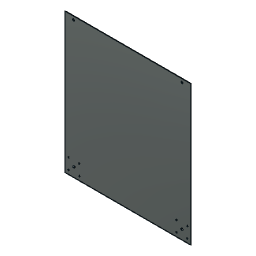
h_bot_Dec26 v12 (Autodesk Fusion 360 design; units mm, degrees)
Autodesk Fusion 360 part; units mm, degrees
sketch "Sketch2" plane through (0, 0, 0) normal (0, 0, 1) x (1, 0, 0)
  line L0 (0, 0) -> (553.4775, 0) construction
  line L1 (0, 0) -> (-537.9839, 0) construction
  line L2 (0, 0) -> (0, 375) construction
  line L3 (0, 0) -> (0, -800) construction
  line L4 (-180, 200) -> (180, 200)
  line L5 (180, 200) -> (180, -200)
  line L6 (180, -200) -> (-180, -200)
  line L7 (-180, -200) -> (-180, 200)
  line L8 (-170, -157.8089) -> (-139, -188.8089) construction
  line L9 (-139, -157.8089) -> (-170, -188.8089) construction
  line L10 (139, -158.0835) -> (170, -189.0835) construction
  line L11 (170, -158.0835) -> (139, -189.0835) construction
  circle A0 centre (-154.5, -173.3089) radius 8
  circle A1 centre (154.5, -173.5835) radius 8
  circle A2 centre (139, -158.0835) radius 1.75
  circle A3 centre (139, -189.0835) radius 1.75
  circle A4 centre (170, -189.0835) radius 1.75
  circle A5 centre (170, -158.0835) radius 1.75
  line L12 (-108, 159) -> (108, 159)
  line L13 (108, 159) -> (108, -120)
  line L14 (108, -120) -> (-108, -120)
  line L15 (-108, -120) -> (-108, 159)
  line L16 (154.5, -173.5835) -> (154.5, 269.9863) construction
  line L17 (-155.5, -173.9681) -> (-155.5, 269.9863) construction
  line L18 (-319.8669, 190) -> (350, 190) construction
  circle A6 centre (-155.5, 190) radius 11.5
  circle A7 centre (154.5, 190) radius 11.5
  circle A8 centre (-155.5, 190) radius 2.5
  circle A9 centre (154.5, 190) radius 2.5
  line L19 (-144, 190) -> (-144, -80) construction
  line L20 (143, 190) -> (143, -60) construction
  circle A10 centre (-170, -157.8089) radius 1.75
  circle A11 centre (-139, -157.8089) radius 1.75
  circle A12 centre (-170, -188.8089) radius 1.75
  circle A13 centre (-139, -188.8089) radius 1.75
  circle A14 centre (-154.5, -173.3089) radius 2.75
  circle A15 centre (154.5, -173.5835) radius 2.75
  point P0 (-170, -188.8089)
  point P1 (-139, -188.8089)
  point P2 (-139, -157.8089)
  point P3 (-170, -157.8089)
  point P4 (125, -200)
  point P5 (170, -158.0835)
  point P6 (139, -189.0835)
  point P7 (139, -158.0835)
  point P8 (170, -189.0835)
  dimension "d11" = 360
  dimension "d12" = 400
  dimension "d36" = 31
  dimension "d37" = 31
  dimension "d38" = 10
  dimension "d39" = 31
  dimension "d40" = 31
  dimension "d41" = 10
  dimension "d42" = 16
  dimension "d43" = 16
  dimension "d44" = 3.5
  dimension "d46" = 3.5
  dimension "d47" = 3.5
  dimension "d48" = 3.5
  dimension "d49" = 279
  dimension "d50" = 216
  dimension "d51" = 80
  dimension "d52" = 10
  dimension "d53" = 23
  dimension "d54" = 23
  dimension "d55" = 5
  dimension "d56" = 5
  dimension "d57" = 24.5
  dimension "d68" = 3.5
  dimension "d69" = 3.5
  dimension "d70" = 3.5
  dimension "d71" = 3.5
  dimension "d72" = 5.5
  dimension "d73" = 5.5
  constraint coincident L0.start L1.start
  constraint horizontal L0
  constraint parallel L0 L1
  constraint perpendicular L0 L2
  constraint perpendicular L0 L3
  constraint horizontal L4
  constraint vertical L5
  constraint horizontal L6
  constraint vertical L7
  constraint symmetric L1 L4 L6
  constraint symmetric L2 L5 L7
  constraint vertical P1 P2
  constraint vertical P0 P3
  constraint horizontal P2 P3
  constraint horizontal P0 P1
  constraint coincident P3 L8.start
  constraint coincident P1 L8.end
  constraint coincident P2 L9.start
  constraint coincident P0 L9.end
  constraint vertical P5 P8
  constraint vertical P6 P7
  constraint horizontal P5 P7
  constraint horizontal P6 P8
  constraint coincident P7 L10.start
  constraint coincident P8 L10.end
  constraint coincident P5 L11.start
  constraint coincident P6 L11.end
  constraint midpoint L9 A0.centre
  constraint midpoint L10 A1.centre
  constraint horizontal L12
  constraint vertical L13
  constraint horizontal L14
  constraint vertical L15
  constraint symmetric L2 L13 L15
  constraint coincident A1.centre L16.start
  constraint perpendicular L4 L16
  constraint perpendicular L5 L18
  constraint coincident L18 A6.centre
  constraint coincident L17 A6.centre
  constraint coincident L18 A7.centre
  constraint coincident L16 A7.centre
  constraint concentric A6 A8
  constraint concentric A7 A9
  constraint coincident L18 L19.start
  constraint coincident A6 L19.start
  constraint tangent A6 L19
  constraint coincident L18 L20.start
  constraint coincident A7 L20.start
  constraint tangent A7 L20
  constraint concentric A0 A14
  constraint concentric A1 A15
  measures "d11" distance of L4.start L4.end
  measures "d12" distance of L4.end L5.end
  measures "d36" distance of P0 P1
  measures "d37" distance of P0 P3
  measures "d38" distance of L7 P0
  measures "d39" distance of P6 P8
  measures "d40" distance of P6 P7
  measures "d41" distance of L5 P8
  measures "d42" diameter of A0
  measures "d43" diameter of A1
  measures "d44" diameter of A2
  measures "d46" diameter of A3
  measures "d47" diameter of A4
  measures "d48" diameter of A5
  measures "d49" distance of L12.end L13.end
  measures "d50" distance of L12.start L12.end
  measures "d51" distance of L6 L14
  measures "d52" distance of L4 L18
  measures "d53" diameter of A6
  measures "d54" diameter of A7
  measures "d55" diameter of A8
  measures "d56" diameter of A9
  measures "d57" distance of L7 A6.centre
  measures "d68" diameter of A10
  measures "d69" diameter of A11
  measures "d70" diameter of A12
  measures "d71" diameter of A13
  measures "d72" diameter of A14
  measures "d73" diameter of A15
extrude "Extrude2" add sketch "Sketch2" along normal blind 6 contours L4 L5 L6 L7 A6 A7 | L4 A6 | L4 A7 | A0 | A1 | A2 | A3 | A4 | A5 | L12 L13 L14 L15 | A8 | A9 | A10 | A11 | A12 | A13 | A14 | A15 picked at (-155.5623, 197.4977) picked at (154.4377, 197.4977) makes body 1
sketch "Sketch3" plane through (0, 0, 6) normal (0, 0, 1) x (1, 0, 0)
  line L0 (-180, -200) -> (180, -200)
  line L1 (180, -200) -> (180, 200)
  line L2 (180, 200) -> (-180, 200)
  line L3 (-180, 200) -> (-180, -200)
  line L4 (-150, 37.5) -> (150, 37.5)
  line L5 (150, 37.5) -> (150, -37.5)
  line L6 (150, -37.5) -> (-150, -37.5)
  line L7 (-150, -37.5) -> (-150, 37.5)
  line L8 (0, 0) -> (553.4775, 0)
  line L9 (0, 0) -> (0, 375)
  line L10 (0, 0) -> (-537.9839, 0)
  line L11 (-125, 7.5) -> (125, 7.5)
  line L12 (125, 7.5) -> (125, -7.5)
  line L13 (125, -7.5) -> (-125, -7.5)
  line L14 (-125, -7.5) -> (-125, 7.5)
  circle A0 centre (-132.4183, 22.14) radius 11.5
  circle A1 centre (-132.4183, -22.14) radius 11.5
  circle A2 centre (132.4183, 22.14) radius 11.5
  circle A3 centre (132.4183, -22.14) radius 11.5
  line L15 (0, 0) -> (0, -800)
  circle A4 centre (-132.4183, 22.14) radius 2.5
  circle A5 centre (-132.4183, -22.14) radius 2.5
  circle A6 centre (132.4183, 22.14) radius 2.5
  circle A7 centre (132.4183, -22.14) radius 2.5
  dimension "d19" = 300
  dimension "d20" = 75
  dimension "d24" = 30
  dimension "d26" = 250
  dimension "d58" = 23
  dimension "d59" = 23
  dimension "d60" = 23
  dimension "d61" = 23
  dimension "d62" = 5
  dimension "d63" = 5
  dimension "d64" = 5
  dimension "d65" = 5
  constraint horizontal L4
  constraint vertical L5
  constraint horizontal L6
  constraint vertical L7
  constraint symmetric L4 L6 L8
  constraint symmetric L5 L7 L9
  constraint horizontal L11
  constraint vertical L12
  constraint horizontal L13
  constraint vertical L14
  constraint symmetric L8 L11 L13
  constraint symmetric L9 L12 L14
  constraint symmetric L10 A0 A1
  constraint symmetric L9 A0 A2
  constraint symmetric A1 A3 L15
  constraint concentric A0 A4
  constraint concentric A1 A5
  constraint concentric A2 A6
  constraint concentric A3 A7
  measures "d19" distance of L4.start L4.end
  measures "d20" distance of L4.end L5.end
  measures "d24" distance of L4 L11.start
  measures "d26" distance of L12 L14
  measures "d58" diameter of A0
  measures "d59" diameter of A1
  measures "d60" diameter of A2
  measures "d61" diameter of A3
  measures "d62" diameter of A4
  measures "d63" diameter of A5
  measures "d64" diameter of A6
  measures "d65" diameter of A7
extrude "Extrude3" add sketch "Sketch3" along normal blind 6 separate body contours L5 L6 L8 L12 L13 L15 | L6 L7 L10 L13 L14 L15 | L4 L7 L9 L10 L11 L14 | L4 L5 L8 L9 L11 L12 | A0 | A1 | A2 | A3 | A4 | A5 | A6 | A7 makes body 2
sketch "Sketch4" plane through (0, 0, 12) normal (0, 0, 1) x (1, 0, 0)
  line L0 (-125, -7.5) -> (-125, 7.5)
  line L1 (-125, 7.5) -> (125, 7.5)
  line L2 (125, 7.5) -> (125, -7.5)
  line L3 (-150, -37.5) -> (150, -37.5)
  line L4 (150, -37.5) -> (150, 37.5)
  line L5 (150, 37.5) -> (-150, 37.5)
  line L6 (-150, 37.5) -> (-150, -37.5)
  line L7 (9.5492, 18.75) -> (34.5492, 18.75)
  line L8 (34.5492, 18.75) -> (34.5492, -18.75)
  line L9 (34.5492, -18.75) -> (9.5492, -18.75)
  line L10 (9.5492, -18.75) -> (9.5492, 18.75)
  line L11 (0, 0) -> (-537.9839, 0)
  line L12 (125, -7.5) -> (-125, -7.5)
  dimension "d31" = 37.5
  dimension "d32" = 25
  constraint horizontal L7
  constraint vertical L8
  constraint horizontal L9
  constraint vertical L10
  constraint symmetric L7 L9 L11
  measures "d31" distance of L7.start L9.end
  measures "d32" distance of L8.end L9.end
extrude "Extrude5" add sketch "Sketch3" along normal blind 5 separate body contours L5 L6 L8 L12 L13 L15 | L6 L7 L10 L13 L14 L15 | L4 L7 L9 L10 L11 L14 | L4 L5 L8 L9 L11 L12 | A0 | A1 | A2 | A3 makes body 3
sketch "Sketch5" plane through (0, 0, 11) normal (0, 0, 1) x (1, 0, 0)
  circle A0 centre (-132.4183, 22.14) radius 2.5
  line L0 (125, -7.5) -> (-125, -7.5)
  line L1 (-125, -7.5) -> (-125, 7.5)
  line L2 (-125, 7.5) -> (125, 7.5)
  line L3 (125, 7.5) -> (125, -7.5)
  circle A1 centre (132.4183, 22.14) radius 2.5
  circle A2 centre (-132.4183, -22.14) radius 2.5
  circle A3 centre (132.4183, -22.14) radius 2.5
  line L4 (-150, -37.5) -> (150, -37.5)
  line L5 (150, -37.5) -> (150, 37.5)
  line L6 (150, 37.5) -> (-150, 37.5)
  line L7 (-150, 37.5) -> (-150, -37.5)
extrude "Extrude6" add sketch "Sketch2" along normal blind 1 separate body contours L4 L5 L6 L7 A6 A7 | L4 A6 | L4 A7 | A0 | A1 | L12 L13 L14 L15 picked at (-155.5623, 197.4977) picked at (154.4377, 197.4977) makes body 4
sketch "Sketch7" plane through (0, 0, 1) normal (0, 0, 1) x (1, 0, 0)
  circle A0 centre (-170, -157.8089) radius 1.75
  circle A1 centre (154.5, 190) radius 2.5
  circle A2 centre (154.5, -173.5835) radius 2.75
  circle A3 centre (-154.5, -173.3089) radius 2.75
  circle A4 centre (170, -189.0835) radius 1.75
  circle A5 centre (-155.5, 190) radius 2.5
  circle A6 centre (139, -189.0835) radius 1.75
  circle A7 centre (-170, -188.8089) radius 1.75
  circle A8 centre (-139, -157.8089) radius 1.75
  circle A9 centre (170, -158.0835) radius 1.75
  circle A10 centre (-139, -188.8089) radius 1.75
  circle A11 centre (139, -158.0835) radius 1.75
  line L0 (-180, -200) -> (180, -200)
  line L1 (180, -200) -> (180, 200)
  line L2 (180, 200) -> (-180, 200)
  line L3 (-180, 200) -> (-180, -200)
extrude "Extrude4" [rolled back] along distance 6 taper angle 0
hidden bodies 1 2 3
equation "frame_height = 400 mm"
equation "frame_width = 360 mm"
equation "frame_thickness = 40 mm"
equation "d11 = frame_width"
equation "d12 = frame_height"
equation "y_carriage_height = 75 mm"
equation "y_carriage_width = 300 mm"
equation "d19 = y_carriage_width"
equation "d20 = y_carriage_height"
equation "y_carriage_thickness = 30 mm"
equation "d24 = y_carriage_thickness"
equation "y_carriage_inner_width = 250 mm"
equation "d26 = y_carriage_inner_width"
equation "x_carriage_width = 25 mm"
equation "x_carriage_height = 25 mm"
equation "d31 = x_carriage_height * 1.5"
equation "d32 = x_carriage_width"
equation "spool_diam = 23 mm"
equation "d44 = sh_1"
equation "d46 = sh_1"
equation "d47 = sh_1"
equation "d48 = sh_1"
equation "d53 = spool_diam"
equation "d54 = spool_diam"
equation "d58 = spool_diam"
equation "d59 = spool_diam"
equation "d60 = spool_diam"
equation "d61 = spool_diam"
equation "sh_1 = 3.5 mm"
equation "d68 = sh_1"
equation "d69 = sh_1"
equation "d70 = sh_1"
equation "d71 = sh_1"
